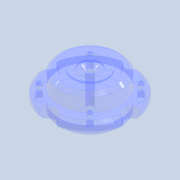
# Autodesk Inventor part: cpd_1.9_p1_v12
Saved by Autodesk Inventor 2021 (Build 250183000, 183)
## iProperties
Created: 2022-10-19
Part Number: cpd_1.9_p1_v12
Material: Generic
Document SubType Name: Modeling
Designer: to172
Density: 1 g/cm^3
Appearance: Clear - Blue
Author: to172
Autodesk Inventor part; units mm, degrees
ref_plane "YZ Plane" through (0, 0, 0) normal (1, 0, 0) x (0, 1, 0)
ref_plane "XZ Plane" through (0, 0, 0) normal (0, 1, 0) x (-1, 0, 0)
ref_plane "XY Plane" through (0, 0, 0) normal (0, 0, 1) x (1, 0, 0)
sketch "Sketch1" plane through (0, 0, 0) normal (0, 0, 1) x (1, 0, 0)
  line L0 (0, 0) -> (0, 19.3687) construction
  line L1 (0, 0) -> (16.1336, 0) construction
  line L2 (9, 11.25) -> (9, 6.25)
  line L3 (9, 6.25) -> (12.5, 6.25)
  line L4 (12.5, 6.25) -> (12.5, 3)
  line L5 (12.5, 3) -> (9, 3)
  line L6 (9, 3) -> (9, 0)
  line L7 (9, 0) -> (1.05, 0)
  line L8 (1.05, 0) -> (1.05, 11.25)
  line L9 (1.05, 11.25) -> (9, 11.25)
  line L10 (3, 11.25) -> (5, 11.25)
  line L11 (5, 11.25) -> (5, 10.75)
  line L12 (5, 10.75) -> (3, 10.75)
  line L13 (3, 10.75) -> (3, 11.25)
  dimension "d0" = 9
  dimension "d1" = 12.5
  dimension "d2" = 1.05
  dimension "d3" = 0.5
  dimension "d4" = 3
  dimension "d5" = 5
  dimension "d6" = 11.25
  dimension "d7" = 5
  dimension "d8" = 3
  constraints: 28 end point, 7 perpendicular, 5 point on line, 2 horizontal, 2 parallel, 1 vertical
  measures "d0" distance between parallel lines of L2 L0
  measures "d1" distance between parallel lines of L4 L0
  measures "d2" distance between parallel lines of L8 L0
  measures "d3" distance between parallel lines of L9 L12
  measures "d4" distance between parallel lines of L13 L0
  measures "d5" distance between parallel lines of L0 L11
  measures "d6" distance between parallel lines of L9 L1
  measures "d7" distance between parallel lines of L3 L9
  measures "d8" distance between parallel lines of L5 L1
revolve "Revolution1" add sketch "Sketch1" angle 360 about axis through (0, 0, 0) along (0, 1, 0) contours L2 L3 L4 L5 L6 L7 L8 L9 L13 L12 L11
sketch "Sketch2" plane through (0, 6.25, 0) normal (0, 1, 0) x (1, 0, 0)
  circle A0 centre (0, 0) radius 12.5 projected
  circle A1 centre (0, 0) radius 12.5 projected
  circle A2 centre (-12.5, 0) radius 2.5
  line L0 (0, 0) -> (-12.5, 0)
  point P0 (-12.25, 2.4875)
  point P1 (-12.25, -2.4875)
  dimension "d10" = 5
  constraints: 2 end point, 1 centre point, 1 horizontal, 1 horizontal alignment, 1 other
  measures "d10" diameter of A2
extrude "Extrusion1" cut sketch "Sketch2" against normal through all contours A2 L0 A0 | A0 L0 A2
pattern_circular "Circular Pattern1" count 4 over 360 about axis through (0, -10, 0) along (0, 1, 0) of "Extrusion1"
chamfer "Chamfer1" distance 1 angle 45 12 edges at (-9, 11.25, 0) (-1.05, 11.25, 0) (-1.05, 0, 0) (-9, 0, 0) (8.8388, 3, 8.8388) (-8.8388, 3, 8.8388) (-8.8388, 3, -8.8388) (8.8388, 3, -8.8388) (8.8388, 6.25, 8.8388) (8.8388, 6.25, -8.8388) (-8.8388, 6.25, -8.8388) (-8.8388, 6.25, 8.8388)
sketch "Sketch3" plane through (0, 3, 12.5) normal (0, -1, 0) x (1, 0, 0)
  line L0 (0, -12.5) -> (0, 1.0988) construction
  line L1 (0, -12.5) -> (-11.9674, -0.5326) construction
  circle A0 centre (-7.4246, -5.0754) radius 0.8
  dimension "d19" = 45
  dimension "d20" = 1.6
  dimension "d21" = 10.5
  constraints: 4 end point, 1 centre point, 1 point on line, 1 vertical
  measures "d19" angle of L0 L1
  measures "d20" diameter of A0
  measures "d21" distance of L0.start A0.centre
extrude "Extrusion2" cut sketch "Sketch3" against normal blind 2
chamfer "Chamfer2" distance 0.25 angle 45 1 edges at (-8.2246, 3, 7.4246)
pattern_circular "Circular Pattern2" count 4 over 360 about axis through (0, -10, 0) along (0, 1, 0) of "Extrusion2", "Chamfer2"
sketch "Sketch4" plane through (0, 6.25, 12.5) normal (0, 1, 0) x (1, 0, 0)
  circle A0 centre (0, 12.5) radius 1.05 construction
  line L0 (0, 12.5) -> (0, -5.5478) construction
  line L1 (0, 12.5) -> (-15.1485, -2.6485) construction
  circle A1 centre (-7.4246, 5.0754) radius 0.75
  dimension "d30" = 45
  dimension "d31" = 1.5
  dimension "d32" = 10.5
  constraints: 4 end point, 1 centre point, 1 point on line, 1 vertical
  measures "d30" angle of L0 L1
  measures "d31" diameter of A1
  measures "d32" distance of point (0, 12.5) A1.centre
extrude "Extrusion3" add sketch "Sketch4" along normal blind 1.5
chamfer "Chamfer3" distance 0.35 angle 45 1 edges at (-8.1746, 7.75, 7.4246)
pattern_circular "Circular Pattern3" count 4 over 360 about axis through (0, -10, 0) along (0, 1, 0) of "Extrusion3", "Chamfer3"
body "Solid1"
